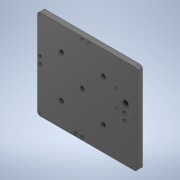
# Autodesk Inventor part: BasePlate
Saved by Autodesk Inventor 2022 (Build 260153000, 153)
## iProperties
Created: 2020-03-15
Part Number: BasePlate
Material: Generic
Document SubType Name: Modeling
Designer: elmar
Density: 1 g/cm^3
Appearance: Smooth - Black
BasePlateCornerRadius: 5.000 mm
BasePlateWidth: 160.000 mm
M3HoleDiameter: 3.200 mm
M3CounterSinkDiameter: 6.300 mm
MountHoleToSideDistance: 5.000 mm
Author: elmar
Autodesk Inventor part; units mm, degrees
ref_plane "YZ Plane" through (0, 0, 0) normal (1, 0, 0) x (0, 1, 0)
ref_plane "XZ Plane" through (0, 0, 0) normal (0, 1, 0) x (-1, 0, 0)
ref_plane "XY Plane" through (0, 0, 0) normal (0, 0, 1) x (1, 0, 0)
sketch "Sketch1" plane through (0, 0, 0) normal (0, 0, 1) x (1, 0, 0)
  line L0 (37.5, -37.5) -> (-37.5, -37.5)
  line L1 (-37.5, -37.5) -> (-37.5, 37.5)
  line L2 (-37.5, 37.5) -> (37.5, 37.5)
  line L3 (37.5, 37.5) -> (37.5, -37.5)
  line L4 (37.5, -37.5) -> (-37.5, 37.5) construction
  line L5 (-37.5, -37.5) -> (37.5, 37.5) construction
  line L6 (-75, 0) -> (0, 75)
  line L7 (0, 75) -> (75, 0)
  line L8 (75, 0) -> (0, -75)
  line L9 (0, -75) -> (-75, 0)
  line L10 (-115.5865, 0) -> (133.519, 0) projected
  circle A0 centre (37.5, 37.5) radius 37.5
  circle A1 centre (76.7825, 15.5482) radius 7.5
  circle A2 centre (37.5, -37.5) radius 38.5
  circle A3 centre (76.7825, 15.5482) radius 9.5
  line L11 (61.2825, 31.0482) -> (92.2825, 31.0482)
  line L12 (92.2825, 31.0482) -> (92.2825, 0.0482)
  line L13 (92.2825, 0.0482) -> (61.2825, 0.0482)
  line L14 (61.2825, 0.0482) -> (61.2825, 31.0482)
  line L15 (97.9325, 36.6982) -> (97.9325, -5.6018)
  line L16 (55.6325, -5.6018) -> (55.6325, 36.6982)
  line L17 (55.6325, 36.6982) -> (97.9325, 36.6982)
  line L18 (-80, 80) -> (97.9325, 80)
  line L19 (97.9325, 80) -> (97.9325, -80)
  line L20 (97.9325, -80) -> (-80, -80)
  line L21 (-80, -80) -> (-80, 80)
  circle A4 centre (76.7825, 15.5482) radius 11.5
  circle A5 centre (75, 0) radius 4.15
  circle A6 centre (61.2825, 0.0482) radius 4.15
  circle A7 centre (37.5, 37.5) radius 4
  line L22 (37.7505, 41.4921) -> (41.4921, 37.7505)
  circle A8 centre (0, 0) radius 4
  line L23 (3.9921, 0.2505) -> (0.2505, 3.9921)
  point P0 (-80, 0)
  dimension "d0" = 75
  dimension "d2" = 75
  dimension "d3" = 15
  dimension "d4" = 77
  dimension "d5" = 19
  dimension "StepperHoleSpacing" = 31
  dimension "StepperWidth" = 42.3
  dimension "StepperCountersinkDiameter" = 23
  dimension "d38" = 8.3
  dimension "d552" = 8.3
  dimension "d554" = 75
  dimension "d555" = 5
  dimension "MountHoleToSideDistance" = 5
  dimension "StepperToEdgeGap" = 0
  dimension "BasePlateWidth" = 160
  dimension "DistanceToCoveredHole" = 24.6421
  dimension "d764" = 8
  dimension "d765" = 3
  constraints: 46 end point, 11 coincident, 9 centre point, 6 parallel, 4 point on circle, 3 midpoint, 3 point on line, 2 equal length, 2 horizontal, 2 perpendicular, 2 tangent, 2 vertical, 1 equal radius, 25 other
  measures "d0" distance of L1.end L2.end
  measures "d2" diameter of A0
  measures "d3" diameter of A1
  measures "d4" diameter of A2
  measures "d5" diameter of A3
  measures "StepperHoleSpacing" distance of L11.start L11.end
  measures "StepperWidth" distance of L16.end L15.start
  measures "StepperCountersinkDiameter" diameter of A4
  measures "d38" diameter of A5
  measures "d552" diameter of A6
  measures "d554" distance of L7.end point (0, 0)
  measures "d555" distance from line of L18 L6.end
  measures "MountHoleToSideDistance" distance from line of L21 L6.start
  measures "StepperToEdgeGap" distance between parallel lines of L15 L19
  measures "BasePlateWidth" distance of L20.end L18.start
  measures "DistanceToCoveredHole" distance of L11.start L2.end
  measures "d764" diameter of A7
  measures "d765" distance between parallel lines of L22 L7
extrude "Extrusion1" add sketch "Sketch1" along normal blind 9 contours L8 A2 L0 | L0 A2 L10 L3 | L3 L10 A2 L8 | L8 A2 | A2 L8 L9 L0 | L0 L1 L10 A8 A2 | A0 A2 L3 | A0 A2 L10 | L10 A2 A0 | L3 A2 A0 | A2 L16 L10 A6 A5 L8 | L8 A5 L10 L15 L19 L20 L21 L9 A2 | L9 L10 L1 | L10 A8 L1 L2 A0 A2 | A2 A0 L2 A7 L3 | L3 A7 L7 L16 A0 A2 | A2 A0 L16 L10 | L10 L16 A2 | A5 L10 L8 | L8 L10 A5 | L10 L6 L1 | L10 L21 L18 L19 L17 A0 L7 L6 | A8 L10 | L10 A8 L23 | A7 L2 L3 | L3 L7 A7 | L16 A0 L14 A6 L10 | A0 L7 A7 L2 | L2 L6 L7 A0 | L16 L7 L14 A0 | L10 A5 L13 L7 | L7 L13 A5 L10 | L10 A6 L13 A5 | A5 L13 L12 L11 A0 L17 L15 L10 | L23 A8 | L2 A7 L7 | L7 A7 L22 | A7 L7 A0 L17 L16 | A6 L14 L13 L10 | L10 A6 | L14 L7 A0 | A0 L7 A5 L13 A6 L14 | L16 L17 A0 L11 L14 L7 | L13 A5 L7 | L7 A5 L13 | A5 A4 A0 L11 L12 L13 | A6 L13 L14 | A0 A4 A5 L7 | L7 L14 L11 A0 A4 | A4 A0 A3 | A7 L22 | A4 A0 A3 | A3 A0 | A1 | A0 A3
fillet "Fillet1" radius 5 4 edges at (-80, 80, 4.5) (97.9325, 80, 4.5) (97.9325, -80, 4.5) (-80, -80, 4.5)
hole "Hole1" at (92.2825, 31.0482, 0) at (61.2825, 31.0482, 0) at (61.2825, 0.0482, 0) at (92.2825, 0.0482, 0) direction (0, 0, 1) diameter 3.2 depth 9 tip angle 118 countersink diameter 6.3 countersink angle 90 clearance for "Flat Head Machine Screw" size "M3" standard "Ansi Metric M Profile"
sketch "Sketch2" plane through (0, 0, 9) normal (0, 0, 1) x (1, 0, 0)
  circle A0 centre (76.7825, 15.5482) radius 11
  line L0 (75, 0) -> (75, -12)
  point P0 (0, 0)
  dimension "d660" = 22
  dimension "d773" = 12
  constraints: 2 coincident, 2 end point, 1 centre point, 1 vertical
  measures "d660" diameter of A0
  measures "d773" distance of L0.start L0.end
hole "Hole2" at (75, 0, 9) at (75, -12, 9) direction (0, 0, -1) diameter 3.2 depth 9 tip angle 118 countersink diameter 6.3 countersink angle 90 clearance for "Flat Head Machine Screw" size "M3" standard "Ansi Metric M Profile"
extrude "Extrusion7" cut sketch "Sketch1" along normal through all contours A7 L2 L3 | L3 L7 A7 | L2 A7 L7 | L7 A7 L22
pattern_circular "Circular Pattern1" count 4 over 360 about axis through (0, 0, -10) along (0, 0, 1) of "Extrusion7"
extrude "Extrusion8" cut sketch "Sketch1" along normal through all contours A8 L10 | L10 A8 L23
sketch "Sketch3" plane through (0, 0, 0) normal (0, 0, -1) x (-1, 0, 0)
  line L0 (-92.9325, 75) -> (75, 75)
  line L1 (75, 75) -> (75, -75)
  line L2 (75, -75) -> (-92.9325, -75)
  line L3 (-92.9325, -75) -> (-92.9325, 75)
  arc A0 (-92.9325, 80) -> (-97.9325, 75) centre (-92.9325, 75) ccw projected
  line L4 (117.6412, 0) -> (-138.5984, 0) projected
  arc A1 (80, 75) -> (75, 80) centre (75, 75) ccw projected
  line L5 (-101.9927, 46.55) -> (-59.6927, 46.55)
  line L6 (-59.6927, 46.55) -> (-59.6927, 4.25)
  line L7 (-59.6927, 4.25) -> (-101.9927, 4.25)
  line L8 (-101.9927, 4.25) -> (-101.9927, 46.55)
  point P0 (0, 0)
  point P1 (-92.9325, 0)
  point P2 (-80.8427, 25.4)
  point P3 (-80.8427, 25.4)
  dimension "d50" = 42.3
  constraints: 16 end point, 3 coincident, 2 horizontal, 2 parallel, 1 midpoint, 1 perpendicular, 1 point on line, 9 other
  measures "d50" distance of L7.end L5.start
hole "Hole4" at (92.9325, 75, 0) at (-75, 75, 0) at (-75, -75, 0) at (92.9325, -75, 0) direction (0, 0, 1) diameter 3.2 depth 9 tip angle 118 countersink diameter 6.3 countersink angle 90 clearance for "Flat Head Machine Screw" size "M3" standard "Ansi Metric M Profile"
hole "Hole7" at (76.7825, 15.5482, 0) direction (0, 0, 1) diameter 10 end through all
pattern_circular "Circular Pattern2" count 4 over 360 about axis through (0, 0, -10) along (0, 0, 1) of "Hole2"
equation "\"M3HoleDiameter\" = 3.2"
equation "\"M3CounterSinkDiameter\" = 6.3"
equation "\"d576\" = 55deg"
equation "\"Sketch57_Pitch\" = 1.25"
equation "\"d594\" = 55deg"
equation "\"Sketch59_Pitch\" = 1.25"
equation "\"d612\" = 55deg"
equation "\"Sketch61_Pitch\" = 1.25"
equation "\"d630\" = 55deg"
equation "\"Sketch63_Pitch\" = 1.25"
equation "\"d648\" = 55deg"
equation "\"Sketch65_Pitch\" = 1.25"
equation "\"d670\" = 55deg"
equation "\"Sketch67_Pitch\" = 1.25"
equation "\"d688\" = 55deg"
equation "\"Sketch69_Pitch\" = 1.25"
equation "\"d706\" = 55deg"
equation "\"Sketch71_Pitch\" = 1.25"
equation "\"d724\" = 55deg"
equation "\"Sketch73_Pitch\" = 1.25"
equation "\"d742\" = 55deg"
equation "\"Sketch75_Pitch\" = 1.25"
